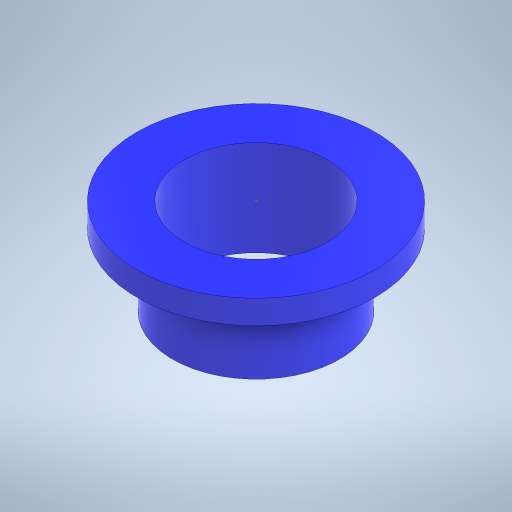
# Autodesk Inventor part: entrada_manguera_2
Saved by Autodesk Inventor 2024 (Build 280153000, 153)
## iProperties
Created: 2022-11-14
Part Number: entrada_manguera_2
Material: Generic
Document SubType Name: Modeling
Designer: ferna
Density: 1 g/cm^3
Appearance: Blue - Wall Paint - Glossy
Author: ferna
Autodesk Inventor part; units mm, degrees
ref_plane "YZ Plane" through (0, 0, 0) normal (1, 0, 0) x (0, 1, 0)
ref_plane "XZ Plane" through (0, 0, 0) normal (0, 1, 0) x (-1, 0, 0)
ref_plane "XY Plane" through (0, 0, 0) normal (0, 0, 1) x (1, 0, 0)
sketch "Sketch1" plane through (0, 0, 0) normal (0, 1, 0) x (-1, 0, 0)
  circle A0 centre (0, 0) radius 3
  circle A1 centre (0, 0) radius 3.5
  dimension "d0" = 6
  dimension "d1" = 7
  constraints: 2 centre point, 2 coincident
  measures "d0" diameter of A0
  measures "d1" diameter of A1
extrude "Extrusion1" add sketch "Sketch1" along normal blind 3
sketch "Sketch2" plane through (0, 3, 0) normal (0, 1, 0) x (1, 0, 0)
  circle A0 centre (0, 0) radius 6.5
  circle A1 centre (0, 0) radius 5
  circle A2 centre (0, 0) radius 3.5 projected
  circle A3 centre (0, 0) radius 3 projected
  dimension "d4" = 13
  constraints: 2 centre point, 2 coincident
  measures "d4" diameter of A0
extrude "Extrusion2" add sketch "Sketch2" along normal blind 1 contours A1 | A2
sketch "Sketch3" plane through (0, 4, 0) normal (0, 1, 0) x (1, 0, 0)
  circle A0 centre (0, 0) radius 3 projected
body "Solid1"
